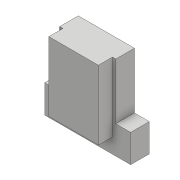
# Autodesk Inventor part: body_bottom
Saved by Autodesk Inventor 2017 (Build 210142000, 142)
## iProperties
Created: 2019-03-28
Part Number: body_bottom
Material: Generic
Document SubType Name: Modeling
Designer: mfans
Density: 1 g/cm^3
Appearance: Default
Author: mfans
Autodesk Inventor part; units mm, degrees
ref_plane "YZ Plane" through (0, 0, 0) normal (1, 0, 0) x (0, 1, 0)
ref_plane "XZ Plane" through (0, 0, 0) normal (0, 1, 0) x (-1, 0, 0)
ref_plane "XY Plane" through (0, 0, 0) normal (0, 0, 1) x (1, 0, 0)
sketch "Sketch1" plane through (0, 0, 0) normal (0, 1, 0) x (-1, 0, 0)
  line L0 (30, 45) -> (-30, 45)
  line L1 (-30, 45) -> (-30, -45)
  line L2 (-30, -45) -> (30, -45)
  line L3 (30, -45) -> (30, 45)
  line L4 (30, 45) -> (-30, -45) construction
  line L5 (-30, 45) -> (30, -45) construction
  point P0 (0, 0)
  dimension "d0" = 90
  dimension "d1" = 60
  constraints: 12 end point, 2 midpoint, 2 parallel, 1 horizontal, 1 perpendicular
  measures "d0" distance of L0.end L1.end
  measures "d1" distance of L1.end L2.end
extrude "Extrusion1" add sketch "Sketch1" along normal blind 20
sketch "Sketch2" plane through (0, 0, 0) normal (0, -1, 0) x (1, 0, 0)
  line L0 (26.5, 45) -> (-26.5, 45)
  line L1 (-26.5, 45) -> (-26.5, -29)
  line L2 (-26.5, -29) -> (26.5, -29)
  line L3 (26.5, -29) -> (26.5, 45)
  line L4 (-30, 45) -> (30, 45) projected
  point P0 (0, 0)
  dimension "d4" = 74
  dimension "d5" = 0
  dimension "d6" = 53
  dimension "d7" = 26.5
  constraints: 8 end point, 2 parallel, 1 horizontal, 1 perpendicular
  measures "d4" distance of L2.end L0.start
  measures "d5" distance between parallel lines of L0 L4
  measures "d6" distance between parallel lines of L3 L1
  measures "d7" distance from line of L1 point (0, 0)
extrude "Extrusion2" add sketch "Sketch2" along normal blind 15
sketch "Sketch3" plane through (30, 0, 45) normal (1, 0, 0) x (0, 0, -1)
  line L0 (0, 0) -> (90, 0) projected
  line L1 (90, 0) -> (90, 20) projected
  line L2 (0, 20) -> (90, 20) projected
  line L3 (0, 0) -> (0, 20) projected
  line L4 (90, 0) -> (60, 0)
  line L5 (60, 0) -> (60, 20)
  line L6 (60, 20) -> (90, 20)
  line L7 (90, 20) -> (90, 0)
  point P0 (45, 0)
  dimension "d10" = 30
  constraints: 8 end point, 2 parallel, 1 horizontal, 1 perpendicular, 1 point on line
  measures "d10" distance between parallel lines of L1 L5
extrude "Extrusion3" add sketch "Sketch3" along normal blind 16 contours L5 L2 L1 L0
mirror "Mirror1" about plane through (0, 0, 0) normal (1, 0, 0) of "Extrusion3"
shell "Shell1" thickness 1 removed faces 1 at (-10, 20, 5)
ref_plane "Work Plane1" through (0, 0, 0) normal (1, 0, 0) x (0, 1, 0)
body "Solid1"
